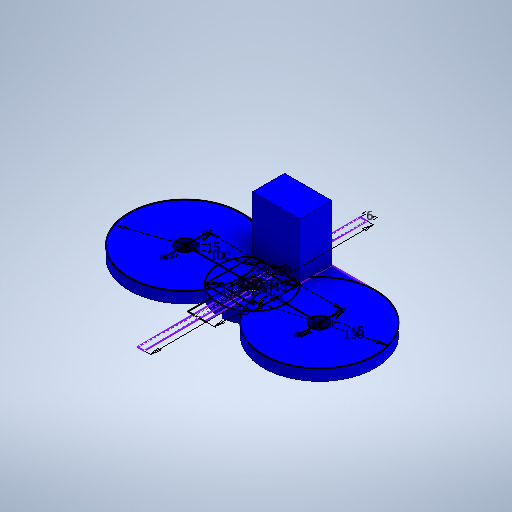
# Autodesk Inventor part: ExtruderFrame
Saved by Autodesk Inventor 2025.2 (Build 292293000, 293)
## iProperties
Created: 2025-05-30
Part Number: ExtruderFrame
Material: Generic
Document SubType Name: Modeling
Designer: Simon
Density: 1 g/cm^3
Appearance: Default(2)
Author: Simon
Autodesk Inventor part; units mm, degrees
ref_plane "YZ Plane" through (0, 0, 0) normal (1, 0, 0) x (0, 1, 0)
ref_plane "XZ Plane" through (0, 0, 0) normal (0, 1, 0) x (-1, 0, 0)
ref_plane "XY Plane" through (0, 0, 0) normal (0, 0, 1) x (1, 0, 0)
sketch "Sketch6" plane through (0, 0, 0) normal (0, 1, 0) x (-1, 0, 0)
  line L0 (60, 0) -> (-60, 0)
  circle A0 centre (0, 0) radius 30
  circle A1 centre (-60, 0) radius 50
  circle A2 centre (60, 0) radius 50
  circle A3 centre (60, 0) radius 7.5
  circle A4 centre (0, 0) radius 7.5
  circle A5 centre (-60, 0) radius 7.5
  line L1 (60, -50) -> (-60, -50)
  line L2 (-60, 18.65) -> (-60, -18.65)
  line L3 (60, 18.65) -> (60, -18.65)
  line L4 (0, -15.3795) -> (0, 15.3795)
  line L5 (15.3795, 15.3795) -> (-15.3795, 15.3795)
  line L6 (15.3795, -15.3795) -> (-15.3795, -15.3795)
  line L7 (21.15, 21.5) -> (-21.15, 21.5)
  line L8 (-21.15, 21.5) -> (-21.15, -21.5)
  line L9 (-21.15, -21.5) -> (21.15, -21.5)
  line L10 (21.15, -21.5) -> (21.15, 21.5)
  line L11 (21.15, 21.5) -> (-21.15, -21.5) construction
  line L12 (-21.15, 21.5) -> (21.15, -21.5) construction
  line L13 (21.15, -21.5) -> (-21.15, -21.5)
  line L14 (-21.15, -21.5) -> (-21.15, -50)
  line L15 (-21.15, -50) -> (21.15, -50)
  line L16 (21.15, -50) -> (21.15, -21.5)
  line L17 (7.5, 0) -> (-7.7, 0)
  line L18 (-7.7, 0) -> (-7.7, 50)
  line L19 (-7.7, 50) -> (7.5, 50)
  line L20 (7.5, 50) -> (7.5, 0)
  line L21 (3.4996, -99.9838) -> (-2.5003, -100.0137)
  line L22 (-2.5003, -100.0137) -> (-3.4996, 99.9838)
  line L23 (-3.4996, 99.9838) -> (2.5003, 100.0137)
  line L24 (2.5003, 100.0137) -> (3.4996, -99.9838)
  line L25 (3.4996, -99.9838) -> (-3.4996, 99.9838) construction
  line L26 (-2.5003, -100.0137) -> (2.5003, 100.0137) construction
  point P0 (16.6667, 24.9444)
  point P1 (-16.6667, 24.9444)
  point P2 (-7.5, 0)
  point P3 (-3, 0)
  point P4 (3, 0)
  point P5 (-21.15, -21.5)
  point P6 (21.15, -50)
  dimension "d39" = 100
  dimension "d40" = 100
  dimension "d42" = 15
  dimension "d37" = 120
  dimension "d38" = 60
  dimension "d41" = 15
  dimension "d43" = 15
  dimension "d46" = 37.3
  dimension "d47" = 37.3
  dimension "d48" = 30.759
  dimension "d49" = 30.759
  dimension "d50" = 30.759
  dimension "d65" = 42.3
  dimension "d66" = 43
  dimension "d67" = 50
  dimension "d70" = 6
  dimension "d71" = 200
  constraints: 54 end point, 10 midpoint, 10 parallel, 6 coincident, 6 horizontal, 4 perpendicular, 3 centre point, 2 point on line, 2 vertical, 9 other
  measures "d37" distance of L0.start L0.end
  measures "d38" diameter of A0
  measures "d41" diameter of A3
  measures "d43" diameter of A5
  measures "d46" distance of L2.start L2.end
  measures "d47" distance of L3.start L3.end
  measures "d48" distance of L4.start L4.end
  measures "d49" distance of L5.start L5.end
  measures "d50" distance of L6.start L6.end
  measures "d65" distance of L9.end L8.end
  measures "d66" distance of L8.end L7.end
  measures "d67" distance of L17.end L18.end
  measures "d70" distance of L21.start L21.end
  measures "d71" distance of L21.end L22.end
extrude "Extrusion8" add sketch "Sketch6" against normal blind 10 contours L0 A4 L22 L6 A1 | L18 L5 L22 A4 L0 | L0 A1 L5 L18 | A1 L9 A0 L8 L0 | L0 L8 A0 L7 A1 | L18 L7 L22 L5 | L5 A1 L7 L18 | L8 A0 L0 | L0 A0 L8 | L6 L22 L9 A1 | L22 L5 L4 A4 | A4 L4 L6 L22 | L22 L7 L24 L5 | L18 A0 L22 L7 | L7 A1 A0 L18 | A0 L8 L14 A1 L7 | L8 L7 A0 | A0 L9 L8 | L7 A0 A1 | L9 L22 A0 A1 | A1 A0 L9 | L6 L24 L9 L22 | L4 L5 L24 A4 | A4 L24 L6 L4 | L22 A0 L24 L7 | A0 A1 L14 L9 | A0 L22 L1 L14 A1 | L9 L24 A0 L22 | L24 L5 L20 A4 | A4 L0 A2 L6 L24 | L24 L7 L20 L5 | L24 A0 L20 L7 | L14 L1 A1 | A0 L24 L1 L22 | L24 L6 A2 L9 | L9 A2 A0 L24 | L20 L5 A2 L0 | L20 L7 A2 L5 | L20 A0 A2 L7 | A0 A2 L16 L1 L24 | L9 A0 A2 | A2 L0 L10 A0 L9 | A2 L7 A0 L10 L0 | A2 A0 L7 | A0 L9 L16 A2 | A0 L10 L9 | L10 A0 L0 | L0 A0 L10 | A2 L16 L10 A0 L7 | L7 L10 A0 | A2 L1 L16
hole "Hole1" at (-15.3795, 0, -15.3795) at (15.3795, 0, -15.3795) at (-15.3795, 0, 15.3795) at (15.3795, 0, 15.3795) direction (0, -1, 0) diameter 3.5 end through all
hole "Hole2" at (-60, 0, -18.65) at (-60, 0, 18.65) at (60, 0, 18.65) at (60, 0, -18.65) direction (0, -1, 0) diameter 5 end through all
extrude "Extrusion10" cut sketch "Sketch6" against normal blind 15 contours L22 A4 L4 L0 | L22 L5 L4 A4 | L22 L7 L24 L5 | L4 A4 L24 L0 | L4 L5 L24 A4 | L22 A0 L24 L7 | L22 L19 L24 A0 | L22 L23 L24 L19 picked at (-2.0114, 2.2863) picked at (1.9885, 2.2963)
extrude "Extrusion11" add sketch "Sketch6" along normal blind 50 contours L9 L22 A0 A1 | A1 A0 L9 | A0 A1 L14 L9 | A0 L22 L1 L14 A1 | L9 L24 A0 L22 | A0 L24 L1 L22 | L9 A2 A0 L24 | A0 A2 L16 L1 L24 | L9 A0 A2 | A0 L9 L16 A2
body "Solid2"
